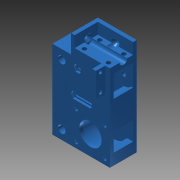
# Autodesk Inventor part: YMotorBlockLeft
Saved by Autodesk Inventor 2015 SP1 (Build 190203100, 203)
## iProperties
Category: Print
Created: 2014-08-14
Part Number: YMotorBlockLeft
Material: ABS Plastic
Document SubType Name: Modeling
Designer: Jack
Density: 1.06 g/cm^3
Appearance: Cyan
Mass: 75.2595 g
Surface Area: 352.616 cm^2
Volume: 70.9995 cm^3
Vendor: Jack
Catalog Web Link: N/A
Author: Jack; Zelogik
Title: Y Motor Block Left
Autodesk Inventor part; units mm, degrees
ref_plane "YZ Plane" through (0, 0, 0) normal (1, 0, 0) x (0, 1, 0)
ref_plane "XZ Plane" through (0, 0, 0) normal (0, 1, 0) x (-1, 0, 0)
ref_plane "XY Plane" through (0, 0, 0) normal (0, 0, 1) x (1, 0, 0)
sketch "Sketch1" plane through (0, 0, 0) normal (0, 1, 0) x (-1, 0, 0)
  line L0 (0, 0) -> (0, -105)
  line L1 (42, 0) -> (0, 0)
  line L2 (0, -105) -> (62, -105)
  line L3 (42, 0) -> (42, -20)
  line L4 (42, -20) -> (62, -20)
  line L5 (62, -20) -> (62, -105)
  dimension "d7" = 105
  dimension "d12" = 62
  dimension "d13" = 20
  dimension "d14" = 20
  constraints: 12 end point, 3 vertical, 2 perpendicular, 1 horizontal, 1 vertical alignment
  measures "d7" distance of L0.start L0.end
  measures "d12" distance of L0.end L2.end
  measures "d13" distance of L1.start L3.end
  measures "d14" distance of L3.end L4.end
extrude "BaseSurface" add sketch "Sketch1" along normal blind 4
sketch "Sketch2" plane through (0, 4, 0) normal (0, 1, 0) x (1, 0, 0)
  line L0 (0, 0) -> (0, 105) projected
  line L1 (0, 105) -> (-62, 105) projected
  line L2 (-62, 105) -> (-62, 20) projected
  line L3 (-62, 20) -> (-42, 20) projected
  line L4 (-42, 20) -> (-42, 0) projected
  line L5 (-42, 0) -> (0, 0) projected
  line L6 (-62, 85) -> (-44.3238, 85)
  line L7 (-6.5778, 93) -> (0, 93)
  line L8 (-8.0385, 73) -> (0, 73)
  line L9 (-10, 71.0385) -> (-10, 46)
  arc A0 (-2, 42.5498) -> (-10, 46) centre (-10, 35) ccw
  line L10 (-2, 42.5498) -> (0, 42.5498)
  arc A1 (-10, 71.0385) -> (-8.0385, 73) centre (-21, 84) ccw
  arc A2 (-6.5778, 93) -> (-36.8602, 90.12) centre (-21, 84) ccw
  arc A3 (-46, 30) -> (-35, 19) centre (-35, 30) ccw
  line L11 (-35, 19) -> (0, 19)
  line L12 (-50, 35) -> (-62, 35)
  line L13 (-46, 30) -> (-46, 31)
  arc A4 (-46, 31) -> (-50, 35) centre (-50, 31) ccw
  arc A5 (-44.3238, 85) -> (-36.8602, 90.12) centre (-44.3238, 93) ccw
  point P0 (-37.9706, 85)
  point P1 (-46, 35)
  dimension "d17" = 21
  dimension "d18" = 21
  dimension "d19" = 20
  dimension "d20" = 12
  dimension "d21" = 32
  dimension "d22" = 10
  dimension "d24" = 35
  dimension "d25" = 10
  dimension "d26" = 2
  dimension "d27" = 17
  dimension "d28" = 17
  dimension "d29" = 11
  dimension "d31" = 30
  dimension "d32" = 27
  dimension "d33" = 15
  dimension "d34" = 11
  dimension "d47" = 4
  dimension "d48" = 8
  constraints: 16 end point, 13 point on circle, 9 point on line, 6 centre point, 6 perpendicular, 6 tangent, 1 horizontal, 1 vertical
  measures "d17" distance from line of L0 A1.centre
  measures "d18" distance from line of L1 A1.centre
  measures "d19" distance between parallel lines of L1 L6
  measures "d20" distance between parallel lines of L1 L7
  measures "d21" distance between parallel lines of L1 L8
  measures "d22" distance between parallel lines of L0 L9
  measures "d24" distance from line of L5 A0.centre
  measures "d25" distance from line of L0 A0.centre
  measures "d26" distance of L10.start L10.end
  measures "d27" radius of A1
  measures "d28" radius of A2
  measures "d29" radius of A0
  measures "d31" distance from line of L5 A3.centre
  measures "d32" distance from line of L2 A3.centre
  measures "d33" distance between parallel lines of L3 L12
  measures "d34" radius of A3
  measures "d47" radius of A4
  measures "d48" radius of A5
extrude "InternalFill" add sketch "Sketch2" along normal blind 21 contours L5 L4 L3 L2 L12 A4 L13 A3 L11 L0 | L10 A0 L9 A1 L8 L0 | L7 A2 A5 L6 L2 L1 L0
sketch "Sketch5" plane through (0, 25, 0) normal (0, 1, 0) x (1, 0, 0)
  line L0 (-42, 20) -> (-42, 0) projected
  line L1 (-42, 0) -> (0, 0) projected
  line L2 (-38, 0) -> (-38, 12)
  line L3 (-38, 12) -> (0, 12)
  line L4 (0, 0) -> (0, 105) projected
  dimension "d43" = 4
  dimension "d44" = 12
  constraints: 4 end point, 2 point on line, 1 perpendicular, 1 vertical
  measures "d43" distance between parallel lines of L0 L2
  measures "d44" distance between parallel lines of L1 L3
extrude "YRodNotch" cut sketch "Sketch5" against normal up to surface (25 mm away)
sketch "Sketch6" plane through (0, 25, 0) normal (0, 1, 0) x (1, 0, 0)
  line L0 (-38, 0) -> (-38, 12) projected
  line L1 (-38, 12) -> (0, 12) projected
  line L2 (-62, 20) -> (-42, 20) projected
  line L3 (-42, 20) -> (-42, 0) projected
  line L4 (-42, 0) -> (-38, 0) projected
  arc A0 (-10, 71.0385) -> (-8.0385, 73) centre (-21, 84) ccw projected
  line L5 (-10, 71.0385) -> (-10, 46) projected
  arc A1 (-2, 42.5498) -> (-10, 46) centre (-10, 35) ccw projected
  line L6 (-2, 42.5498) -> (0, 42.5498) projected
  line L7 (0, 42.5498) -> (0, 73) projected
  line L8 (0, 73) -> (-8.0385, 73) projected
  line L9 (0, 105) -> (-62, 105) projected
  line L10 (-62, 105) -> (-62, 85) projected
  line L11 (-62, 85) -> (-44.3238, 85) projected
  arc A2 (-44.3238, 85) -> (-36.8602, 90.12) centre (-44.3238, 93) ccw projected
  arc A3 (-6.5778, 93) -> (-36.8602, 90.12) centre (-21, 84) ccw projected
  line L12 (-6.5778, 93) -> (0, 93) projected
  line L13 (0, 93) -> (0, 105) projected
  line L14 (-62, 20) -> (-62, 105)
  line L15 (-62, 105) -> (-62, 20) projected
  line L16 (-62, 105) -> (0, 105)
  line L17 (0, 105) -> (0, 12)
  line L18 (0, 12) -> (-38, 12)
  line L19 (0, 12) -> (0, 19) projected
  line L20 (-38, 0) -> (0, 0)
  line L21 (0, 0) -> (0, 12)
  point P0 (-62, 35)
  constraints: 12 end point, 3 collinear, 1 horizontal, 1 perpendicular, 1 vertical
extrude "TopSurface" add sketch "Sketch6" along normal blind 4
sketch "Sketch3" plane through (0, 0, 0) normal (0, -1, 0) x (1, 0, 0)
  arc A0 (-36.8602, -90.12) -> (-6.5778, -93) centre (-21, -84) ccw projected
  arc A1 (-36.8602, -90.12) -> (-6.5778, -93) centre (-21, -84) ccw projected
  circle A2 centre (-21, -84) radius 12
  dimension "d37" = 24
  constraints: 1 centre point, 1 coincident
  measures "d37" diameter of A2
extrude "MotorBulgeCutout" cut sketch "Sketch3" against normal up to surface (4 mm away)
sketch "Sketch7" plane through (0, 29, 0) normal (0, 1, 0) x (1, 0, 0)
  line L0 (0, 0) -> (0, 105) projected
  line L1 (0, 105) -> (-62, 105) projected
  point P0 (0, 10)
  point P1 (-5.5, 68.5)
  point P2 (-5.5, 99.5)
  point P3 (-36.5, 99.5)
  point P4 (-36.5, 68.5)
  dimension "d51" = 31
  dimension "d52" = 31
  dimension "d53" = 5.5
  dimension "d54" = 5.5
  constraints: 2 horizontal alignment, 2 vertical alignment
  measures "d51" distance of point (-36.5, 99.5) point (-36.5, 68.5)
  measures "d52" distance of point (-5.5, 68.5) point (-36.5, 68.5)
  measures "d53" distance from line of L0 point (-5.5, 99.5)
  measures "d54" distance from line of L1 point (-5.5, 99.5)
hole "MotorMountHoles" at (-5.5, 29, -68.5) at (-5.5, 29, -99.5) at (-36.5, 29, -99.5) at (-36.5, 29, -68.5) direction (0, -1, 0) diameter 3.5 end through all counterbore diameter 6.5 counterbore depth 25
sketch "Sketch8" plane through (0, 29, 0) normal (0, 1, 0) x (1, 0, 0)
  arc A0 (-2, 42.5498) -> (-10, 46) centre (-10, 35) ccw projected
  arc A1 (-46, 30) -> (-35, 19) centre (-35, 30) ccw projected
  arc A2 (-46, 30) -> (-35, 19) centre (-35, 30) ccw projected
hole "IdlerBearingHoles" at (-35, 29, -30) at (-10, 29, -35) direction (0, -1, 0) diameter 4.5 end through all counterbore diameter 8 counterbore depth 1.5
sketch "Sketch9" plane through (0, 0, 0) normal (0, -1, 0) x (1, 0, 0)
  circle A0 centre (-35, -30) radius 2.25 projected
  circle A1 centre (-10, -35) radius 2.25 projected
  line L0 (-12.1362, -38.7) -> (-14.2724, -35)
  line L1 (-14.2724, -35) -> (-12.1362, -31.3)
  line L2 (-12.1362, -31.3) -> (-7.8638, -31.3)
  line L3 (-7.8638, -31.3) -> (-5.7276, -35)
  line L4 (-5.7276, -35) -> (-7.8638, -38.7)
  line L5 (-7.8638, -38.7) -> (-12.1362, -38.7)
  line L6 (-32.8638, -33.7) -> (-37.1362, -33.7)
  line L7 (-37.1362, -33.7) -> (-39.2724, -30)
  line L8 (-39.2724, -30) -> (-37.1362, -26.3)
  line L9 (-37.1362, -26.3) -> (-32.8638, -26.3)
  line L10 (-32.8638, -26.3) -> (-30.7276, -30)
  line L11 (-30.7276, -30) -> (-32.8638, -33.7)
  point P0 (0, 0)
  dimension "d69" = 7.4
  constraints: 24 end point, 2 coincident, 2 horizontal, 1 equal length, 26 other
  measures "d69" distance between parallel lines of L4 L1
extrude "IdlerBearingNutTrap" cut sketch "Sketch9" against normal blind 2.5
sketch "Sketch10" plane through (0, 29, 0) normal (0, 1, 0) x (1, 0, 0)
  line L0 (0, 105) -> (-62, 105) projected
  line L1 (-62, 105) -> (-62, 20) projected
  line L2 (-23, 56.5) -> (-38, 56.5) construction
  line L3 (-23, 58.75) -> (-38, 58.75)
  line L4 (-38, 54.25) -> (-23, 54.25)
  arc A0 (-23, 54.25) -> (-23, 58.75) centre (-23, 56.5) ccw
  arc A1 (-38, 58.75) -> (-38, 54.25) centre (-38, 56.5) ccw
  point P0 (-30.5, 56.5)
  dimension "d72" = 15
  dimension "d73" = 4.5
  dimension "d74" = 48.5
  dimension "d75" = 24
  constraints: 8 end point, 4 point on circle, 4 tangent, 2 centre point, 1 horizontal, 1 midpoint, 1 parallel
  measures "d72" distance of L2.start L2.end
  measures "d73" diameter of A1
  measures "d74" distance from line of L0 L2.end
  measures "d75" distance from line of L1 L2.end
extrude "TensionerBearingSlot" cut sketch "Sketch10" against normal up to surface (29 mm away)
sketch "Sketch11" plane through (0, 29, 0) normal (0, 1, 0) x (1, 0, 0)
  line L0 (-38, 58.75) -> (-23, 58.75) projected
  arc A0 (-23, 54.25) -> (-23, 58.75) centre (-23, 56.5) ccw projected
  line L1 (-23, 54.25) -> (-38, 54.25) projected
  arc A1 (-38, 58.75) -> (-38, 54.25) centre (-38, 56.5) ccw projected
  line L2 (-23, 56.5) -> (-38, 56.5) construction
  line L3 (-23, 60.5) -> (-38, 60.5)
  line L4 (-38, 52.5) -> (-23, 52.5)
  arc A2 (-23, 52.5) -> (-23, 60.5) centre (-23, 56.5) ccw
  arc A3 (-38, 60.5) -> (-38, 52.5) centre (-38, 56.5) ccw
  point P0 (-30.5, 56.5)
  dimension "d78" = 8
  constraints: 8 end point, 4 point on circle, 4 tangent, 2 centre point, 1 horizontal, 1 midpoint, 1 parallel
  measures "d78" diameter of A3
extrude "TensionerBearingHeadSlot" cut sketch "Sketch11" against normal blind 1.5
sketch "Sketch12" plane through (0, 0, 0) normal (0, -1, 0) x (1, 0, 0)
  arc A0 (-38, -54.25) -> (-38, -58.75) centre (-38, -56.5) ccw projected
  arc A1 (-23, -58.75) -> (-23, -54.25) centre (-23, -56.5) ccw projected
  line L0 (-18.7276, -56.5) -> (-20.8638, -60.2)
  line L1 (-20.8638, -60.2) -> (-25.1362, -60.2)
  line L2 (-25.1362, -60.2) -> (-27.2724, -56.5)
  line L3 (-27.2724, -56.5) -> (-25.1362, -52.8)
  line L4 (-25.1362, -52.8) -> (-20.8638, -52.8)
  line L5 (-20.8638, -52.8) -> (-18.7276, -56.5)
  line L6 (-42.2724, -56.5) -> (-40.1362, -52.8)
  line L7 (-40.1362, -52.8) -> (-35.8638, -52.8)
  line L8 (-35.8638, -52.8) -> (-33.7276, -56.5)
  line L9 (-33.7276, -56.5) -> (-35.8638, -60.2)
  line L10 (-35.8638, -60.2) -> (-40.1362, -60.2)
  line L11 (-40.1362, -60.2) -> (-42.2724, -56.5)
  line L12 (-35.8638, -52.8) -> (-25.1362, -52.8)
  line L13 (-25.1362, -60.2) -> (-35.8638, -60.2)
  point P0 (0, 0)
  dimension "d201" = 7.4
  constraints: 28 end point, 2 coincident, 2 horizontal, 1 horizontal alignment, 26 other
  measures "d201" distance between parallel lines of L1 L4
extrude "TensionerBearingNutSlot" cut sketch "Sketch12" against normal blind 2.5
sketch "Sketch13" plane through (0, 0, 0) normal (0, -1, 0) x (1, 0, 0)
  line L0 (-62, -20) -> (-42, -20) projected
  line L1 (-62, -105) -> (-62, -20) projected
  line L2 (0, -105) -> (-62, -105) projected
  point P0 (0, 0)
  point P1 (-52, -30)
  point P2 (-52, -95)
  dimension "d84" = 10
  dimension "d85" = 10
  dimension "d86" = 10
  constraints: 1 vertical alignment
  measures "d84" distance from line of L1 point (-52, -30)
  measures "d85" distance from line of L0 point (-52, -30)
  measures "d86" distance from line of L2 point (-52, -95)
hole "FrameMountHolesBack" at (-52, 0, -30) at (-52, 0, -95) direction (0, 1, 0) diameter 4.5 end through all counterbore diameter 8 counterbore depth 25
sketch "Sketch14" plane through (0, 0, -12) normal (1, 0, 0) x (0, 0, -1)
  line L0 (-12, 29) -> (93, 29) projected
  line L1 (0, 25) -> (0, 0) projected
  circle A0 centre (0, 14.5) radius 4.1
  point P0 (-12, 0)
  dimension "d94" = 8.2
  dimension "d96" = 14.5
  constraints: 1 centre point, 1 point on line
  measures "d94" diameter of A0
  measures "d96" distance from line of L0 A0.centre
extrude "YRodHole" cut sketch "Sketch14" against normal up to surface (38 mm away)
sketch "Sketch43" plane through (-38, 0, 0) normal (1, 0, 0) x (0, 0, -1)
  line L0 (0, 0) -> (0, 25) projected
  arc A0 (12, 10.4) -> (12, 18.6) centre (12, 14.5) ccw projected
  circle A1 centre (10, 14.5) radius 2.25
  dimension "d218" = 4.5
  dimension "d219" = 10
  constraints: 1 centre point, 1 horizontal alignment
  measures "d218" diameter of A1
  measures "d219" distance from line of L0 A1.centre
extrude "Extrusion35" cut sketch "Sketch43" against normal up to surface (4 mm away)
sketch "Sketch44" plane through (-38, 0, -12) normal (0, 0, 1) x (1, 0, 0)
  line L0 (0, 10.4) -> (0, 0) projected
  line L1 (38, 0) -> (0, 0) projected
  line L2 (38, 10.4) -> (38, 0) projected
  line L3 (0, 18.6) -> (38, 18.6) projected
  line L4 (38, 25) -> (38, 18.6) projected
  line L5 (0, 25) -> (38, 25) projected
  line L6 (0, 25) -> (0, 18.6) projected
  circle A0 centre (6, 4.5) radius 2.25
  circle A1 centre (32, 4.5) radius 2.25
  circle A2 centre (6, 21) radius 2.25
  circle A3 centre (32, 21) radius 2.25
  dimension "d226" = 6
  dimension "d227" = 6
  dimension "d228" = 4.5
  dimension "d229" = 4
  dimension "d259" = 4.5
  constraints: 4 centre point, 3 equal radius, 2 horizontal alignment, 2 vertical alignment
  measures "d226" distance from line of L0 A0.centre
  measures "d227" distance from line of L2 A1.centre
  measures "d228" distance from line of L1 A0.centre
  measures "d229" distance from line of L5 A2.centre
  measures "d259" diameter of A2
extrude "Extrusion36" cut sketch "Sketch44" against normal up to surface (7 mm away) contours A0 | A1 | A2 | A3
sketch "Sketch45" plane through (0, 25, 0) normal (0, -1, 0) x (1, 0, 0)
  line L0 (-38, 0) -> (-38, -12) projected
  line L1 (-38, 0) -> (0, 0) projected
  circle A0 centre (-19, -10) radius 2.25
  dimension "d232" = 4.5
  dimension "d233" = 19
  dimension "d234" = 10
  constraints: 1 centre point
  measures "d232" diameter of A0
  measures "d233" distance from line of L0 A0.centre
  measures "d234" distance from line of L1 A0.centre
extrude "Extrusion37" cut sketch "Sketch45" against normal up to surface (4 mm away)
ref_plane "Work Plane3" through (-19, 0, 0) normal (1, 0, 0) x (0, 0, -1)
sketch "Sketch46" plane through (-19, 0, 0) normal (1, 0, 0) x (0, 0, -1)
  line L0 (12, 25) -> (7.75, 25) projected
  line L1 (7.75, 29) -> (12.25, 29) projected
  line L2 (12, 25) -> (12, 25) projected
  line L3 (12, 25) -> (12, 25) projected
  line L4 (0, 25) -> (12, 25) projected
  line L5 (10, 25) -> (5.75, 25)
  line L6 (5.75, 25) -> (7.75, 27.5)
  line L7 (7.75, 27.5) -> (10, 27.5)
  line L8 (10, 27.5) -> (10, 25)
  point P0 (0, 0)
  point P1 (10, 29)
  dimension "d238" = 4.25
  dimension "d239" = 2.5
  constraints: 8 end point, 2 point on line, 2 vertical alignment, 1 midpoint, 1 parallel, 1 perpendicular
  measures "d238" distance of L5.start L5.end
  measures "d239" distance between parallel lines of L0 L7
revolve "Revolution6" cut sketch "Sketch46" angle 360 about axis through (-19, 27.5, -10) along (0, -1, 0)
sketch "Sketch47" plane through (0, 25, 0) normal (0, -1, 0) x (1, 0, 0)
  arc A0 (-15.25, -12) -> (-22.75, -12) centre (-19, -10) ccw projected
  arc A1 (-22.75, -12) -> (-15.25, -12) centre (-19, -10) ccw projected
  circle A2 centre (-19, -10) radius 2.25 projected
extrude "Extrusion38" cut sketch "Sketch47" along normal blind 6 contours A1 A0 | A2
sketch "Sketch48" plane through (0, 25, -19) normal (0, 0, -1) x (-1, 0, 0)
  arc A0 (34.1937, -21) -> (29.8063, -21) centre (32, -20.5) ccw projected
  arc A1 (8.1937, -21) -> (3.8063, -21) centre (6, -20.5) ccw projected
  circle A2 centre (6, -4) radius 2.25 projected
  circle A3 centre (32, -4) radius 2.25 projected
  line L0 (10.2724, -4) -> (8.1362, -7.7)
  line L1 (8.1362, -7.7) -> (3.8638, -7.7)
  line L2 (3.8638, -7.7) -> (1.7276, -4)
  line L3 (1.7276, -4) -> (3.8638, -0.3)
  line L4 (3.8638, -0.3) -> (8.1362, -0.3)
  line L5 (8.1362, -0.3) -> (10.2724, -4)
  line L6 (10.2724, -20.5) -> (8.1362, -24.2)
  line L7 (8.1362, -24.2) -> (3.8638, -24.2)
  line L8 (3.8638, -24.2) -> (1.7276, -20.5)
  line L9 (1.7276, -20.5) -> (3.8638, -16.8)
  line L10 (3.8638, -16.8) -> (8.1362, -16.8)
  line L11 (8.1362, -16.8) -> (10.2724, -20.5)
  line L12 (27.7276, -20.5) -> (29.8638, -16.8)
  line L13 (29.8638, -16.8) -> (34.1362, -16.8)
  line L14 (34.1362, -16.8) -> (36.2724, -20.5)
  line L15 (36.2724, -20.5) -> (34.1362, -24.2)
  line L16 (34.1362, -24.2) -> (29.8638, -24.2)
  line L17 (29.8638, -24.2) -> (27.7276, -20.5)
  line L18 (27.7276, -4) -> (29.8638, -0.3)
  line L19 (29.8638, -0.3) -> (34.1362, -0.3)
  line L20 (34.1362, -0.3) -> (36.2724, -4)
  line L21 (36.2724, -4) -> (34.1362, -7.7)
  line L22 (34.1362, -7.7) -> (29.8638, -7.7)
  line L23 (29.8638, -7.7) -> (27.7276, -4)
  point P0 (0, -25)
  dimension "d243" = 7.4
  constraints: 48 end point, 4 coincident, 4 horizontal, 3 equal length, 52 other
  measures "d243" distance between parallel lines of L16 L13
extrude "Extrusion39" cut sketch "Sketch48" along normal blind 4 and the other way blind 4
ref_plane "Work Plane4" through (-42, 0, -10) normal (0, 0, 1) x (1, 0, 0)
sketch "Sketch49" plane through (-42, 0, -10) normal (0, 0, 1) x (1, 0, 0)
  line L0 (0, 12.25) -> (0, 16.75) projected
  line L1 (4, 16.75) -> (4, 12.25) projected
  line L2 (4, 10.4) -> (4, 18.6) projected
  line L3 (4, 14.5) -> (4, 18.75)
  line L4 (4, 25) -> (4, 18.6) projected
  line L5 (4, 18.75) -> (1.5, 16.75)
  line L6 (1.5, 16.75) -> (1.5, 14.5)
  line L7 (1.5, 14.5) -> (4, 14.5)
  point P0 (42, 0)
  dimension "d249" = 4.25
  dimension "d250" = 2.5
  constraints: 8 end point, 1 horizontal alignment, 1 midpoint, 1 parallel, 1 perpendicular, 1 point on line
  measures "d249" distance of L3.start L3.end
  measures "d250" distance between parallel lines of L1 L6
revolve "Revolution7" cut sketch "Sketch49" angle 360 about axis through (-40.5, 14.5, -10) along (1, 0, 0)
sketch "Sketch51" plane through (0, 4, 0) normal (0, 1, 0) x (1, 0, 0)
  circle A0 centre (-35, 30) radius 2.25 projected
  circle A1 centre (-35, 30) radius 4.75
  point P0 (0, 0)
  dimension "d254" = 9.5
  constraints: 1 centre point, 1 coincident
  measures "d254" diameter of A1
extrude "Extrusion41" cut sketch "Sketch51" against normal blind 0.25
ref_plane "Work Plane5" through (-5.1, 0, -12) normal (1, 0, 0) x (0, 0, -1)
sketch "Sketch53" plane through (-5.1, 0, -12) normal (1, 0, 0) x (0, 0, -1)
  line L0 (0, 0) -> (93, 0) projected
  line L1 (0, 10.4) -> (0, 0) projected
  line L2 (0, 0) -> (0, -10)
  line L3 (0, -10) -> (26.7, -10)
  line L4 (26.7, -10) -> (26.7, 0)
  point P0 (-12, 0)
  dimension "d261" = 10
  dimension "d262" = 26.7
  constraints: 6 end point, 2 perpendicular, 1 point on line, 1 vertical
  measures "d261" distance of L0.start L2.end
  measures "d262" distance of L2.end L3.end
extrude "Extrusion43" add sketch "Sketch53" against normal blind 4
sketch "Sketch54" plane through (-5.1, 0, -12) normal (1, 0, 0) x (0, 0, -1)
  line L0 (26.7, 0) -> (93, 0) projected
  line L1 (26.7, 0) -> (26.7, -10) projected
  circle A0 centre (3.75, -5) radius 1.75
  circle A1 centre (22.75, -5) radius 1.75
  line L2 (0, -10) -> (0, 10.4) projected
  point P0 (-12, 0)
  point P1 (0, 0)
  dimension "d265" = 3.5
  dimension "d266" = 5
  dimension "d268" = 3.95
  dimension "d274" = 3.75
  constraints: 2 centre point, 1 equal radius, 1 horizontal alignment
  measures "d265" diameter of A0
  measures "d266" distance from line of L0 A0.centre
  measures "d268" distance from line of L1 A1.centre
  measures "d274" distance from line of L2 A0.centre
extrude "Extrusion44" cut sketch "Sketch54" against normal up to next
sketch "Sketch55" plane through (-9.1, 0, -12) normal (-1, 0, 0) x (0, 0, 1)
  circle A0 centre (-3.75, -5) radius 1.75 projected
  circle A1 centre (-22.75, -5) radius 1.75 projected
  line L0 (-21.0757, -2.1) -> (-19.4014, -5)
  line L1 (-19.4014, -5) -> (-21.0757, -7.9)
  line L2 (-21.0757, -7.9) -> (-24.4243, -7.9)
  line L3 (-24.4243, -7.9) -> (-26.0986, -5)
  line L4 (-26.0986, -5) -> (-24.4243, -2.1)
  line L5 (-24.4243, -2.1) -> (-21.0757, -2.1)
  line L6 (-2.0757, -2.1) -> (-0.4014, -5)
  line L7 (-0.4014, -5) -> (-2.0757, -7.9)
  line L8 (-2.0757, -7.9) -> (-5.4243, -7.9)
  line L9 (-5.4243, -7.9) -> (-7.0986, -5)
  line L10 (-7.0986, -5) -> (-5.4243, -2.1)
  line L11 (-5.4243, -2.1) -> (-2.0757, -2.1)
  point P0 (12, 0)
  dimension "d271" = 5.8
  constraints: 24 end point, 2 coincident, 2 horizontal, 1 parallel, 26 other
  measures "d271" distance between parallel lines of L4 L1
extrude "Extrusion45" cut sketch "Sketch55" against normal blind 2.5
sketch "Sketch56" plane through (-9.1, 0, -31.3) normal (0, 1, 0) x (1, 0, 0)
  line L0 (0, 0) -> (1.2362, 0) projected
  line L1 (1.2362, 0) -> (3.3724, 3.7) projected
  line L2 (3.3724, 3.7) -> (1.2362, 7.4) projected
  line L3 (1.2362, 7.4) -> (0, 7.4) projected
  line L4 (0, 0) -> (0, 7.4) projected
  point P0 (9.1, -31.3)
extrude "Extrusion46" cut sketch "Sketch56" against normal blind 1
sketch "Sketch57" plane through (-9.1, -1, -31.3) normal (0, 1, 0) x (1, 0, 0)
  line L0 (1.2362, 0) -> (0, 0) projected
  line L1 (3.3724, 3.7) -> (1.2362, 0) projected
  line L2 (1.2362, 7.4) -> (3.3724, 3.7) projected
  line L3 (0, 7.4) -> (1.2362, 7.4) projected
  line L4 (0, 0) -> (0, 7.4) projected
  point P0 (9.1, -31.3)
extrude "Extrusion47" cut sketch "Sketch57" against normal blind 2.5
body "Solid1"
